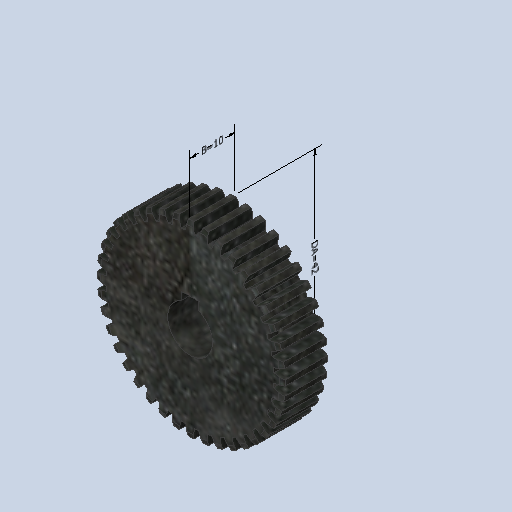
# Autodesk Inventor part: HCWGT-1.0-A-40-10-10
Saved by Autodesk Inventor 2023 (Build 270158000, 158)
## iProperties
Category: PARTsolutions
Company: TOHATSU
Created: 2023-07-27
Part Number: HCWGT-1.0-A-40-10-10
Material: Steel
Catalog Web Link: www.cadenas.de
Description: HCWG-1.0-A-Gear-Module 1.0-A Type
Vendor: TOHATSU
Document SubType Name: Modeling
Designer: psAdmin
Manufacturer: TOHATSU
Mass: 91.3567 g
Surface Area: 53.3619 cm^2
Volume: 11.6378 cm^3
Density: 7.85 g/cm^3
Appearance: Plate
PSOL_IDENT_0: {$CADENAS_DATA/23d-libs/tohatsu/automation_standard_parts/driving_part/toothed_wheel/hcwgt_a_1_0.prj
PSOL_IDENT_1: },195 {VTYP=3D},{NB=HCWGT-1.0-A-40-10-10},{LINA=HCWGT-1.0-A-40-10-10},{NN=HCWG-1.0-A},{DATE=19.07.20
PSOL_IDENT_2: 23 02:54:23},{GEOMDATE=06.12.2022 04:58:41},{VERSION=},{LINEID=10},{WBVAR=TYPE,T,D},{WBNUMERIC=T,D}
PSOL_IDENT_3: {NB=HCWGT-1.0-A-40-10-10},{LINA=HCWGT-1.0-A-40-10-10},{KT=DUMMY},{PN=HCWGT-1.0-A-40-10-10},{ROHS=YE
PSOL_IDENT_4: S},{TYPE=HCWGT},{QU=7850},{MA=S45C},{ST=-},{PR=20°},{CO=0.73,0.75,0.79,0.00},{MO=1.0},{CAMO=1.0},{Y=
PSOL_IDENT_5: A},{T=40},{B=10},{D=10},{DMIN=8},{DMAX=20},{DP=40.0},{DF=37.5},{DA=42.0},{TT=1.57080},{TP=3.14160},{
PSOL_IDENT_6: URL=https://www.tohatsu.com.tw},{WED=網站}
NB: HCWGT-1.0-A-40-10-10
NN: HCWG-1.0-A
NT: Gear-Module 1.0-A Type
NBSYN: $PN.
LINA: HCWGT-1.0-A-40-10-10
CATALOG: TOHATSU
PN: HCWGT-1.0-A-40-10-10
ROHS: YES
TYPE: HCWGT
MA: S45C
ST: -
PR: 20°
MO: 1.0
Y: A
T: 40
B: 10
D: 10
DP: 40
WED: 網站
SUPPLIER: TOHATSU
ARTICLENO: HCWGT-1.0-A-40-10-10
BOMINFO: HCWGT-1.0-A-40-10-10
CREATOR: CADENAS GmbH
Title: HCWGT-1.0-A-40-10-10
Author: Cadenas PARTsolutions
Comments: Gear-Module 1.0-A Type
Autodesk Inventor part; units mm, degrees
ref_plane "YZ Plane" through (0, 0, 0) normal (1, 0, 0) x (0, 1, 0)
ref_plane "XZ Plane" through (0, 0, 0) normal (0, 1, 0) x (-1, 0, 0)
ref_plane "XY Plane" through (0, 0, 0) normal (0, 0, 1) x (1, 0, 0)
sketch "__1" plane through (0, 0, 0) normal (0, 0, 1) x (1, 0, 0)
  circle A0 centre (0, 0) radius 18.75
  constraints: 1 centre point
extrude "Extrusion1" add sketch "__1" along normal blind 10
sketch "__2" plane through (0, 0, 0) normal (0, 0, 1) x (1, 0, 0)
  line L0 (-1.0079, 15.75) -> (1.0079, 15.75)
  line L1 (1.0079, 15.75) -> (1.0079, 18.7229)
  line L2 (1.0079, 18.7229) -> (0.6079, 20.9912)
  arc A0 (0.6079, 20.9912) -> (-0.6079, 20.9912) centre (0, 0) ccw
  line L3 (-0.6079, 20.9912) -> (-1.0079, 18.7229)
  line L4 (-1.0079, 18.7229) -> (-1.0079, 15.75)
  constraints: 10 end point, 2 point on circle, 1 centre point
extrude "Extrusion2" add sketch "__2" along normal blind 10
pattern_circular "Circular Pattern1" count 40 over 360 about axis through (0, 0, 0) along (0, 0, 1) of "Extrusion2"
sketch "__4" plane through (0, 0, 0) normal (1, 0, 0) x (0, 1, 0)
  line L0 (0, -20) -> (0, 20)
  line L1 (26.5, 10) -> (20, 10)
  line L2 (20, 10) -> (21.5, 9.5981)
  line L3 (21.5, 9.5981) -> (21.5, 0.4019)
  line L4 (21.5, 0.4019) -> (20, 0)
  line L5 (20, 0) -> (26.5, 0)
  line L6 (26.5, 0) -> (26.5, 10)
  constraints: 14 end point
sketch "Sketch4" plane through (0, 0, 0) normal (0, 0, -1) x (-1, 0, 0)
  point P0 (0, 0)
hole "Hole1" at (0, 0, 0) direction (0, 0, 1) diameter 10 depth 10
revolve "Revolution1" cut sketch "__4" angle 360 about axis through (0, 0, -20) along (0, 0, -1)
sketch "Sketch5" plane through (0, 0, 10) normal (0, 0, 1) x (1, 0, 0)
  line L0 (-2, 6.4) -> (2, 6.4)
  line L1 (2, 6.4) -> (2, 3.6)
  line L2 (2, 3.6) -> (-2, 3.6)
  line L3 (-2, 3.6) -> (-2, 6.4)
  circle A0 centre (0, 0) radius 5 projected
  line L4 (-2, 6.4) -> (2, 3.6) construction
  line L5 (2, 6.4) -> (-2, 3.6) construction
  point P0 (0, 5)
  dimension "d18" = 4
  dimension "d19" = 1.4
  constraints: 12 end point, 2 midpoint, 2 parallel, 1 horizontal, 1 perpendicular, 1 vertical alignment, 1 other
  measures "d18" distance of L0.start L0.end
  measures "d19" distance from line of L0 point (0, 5)
extrude "Extrusion3" cut sketch "Sketch5" against normal through all contours L0 L1 A0 L3 | A0 L1 L2 L3 picked at (0, 4.0667)
body "Solid1"
